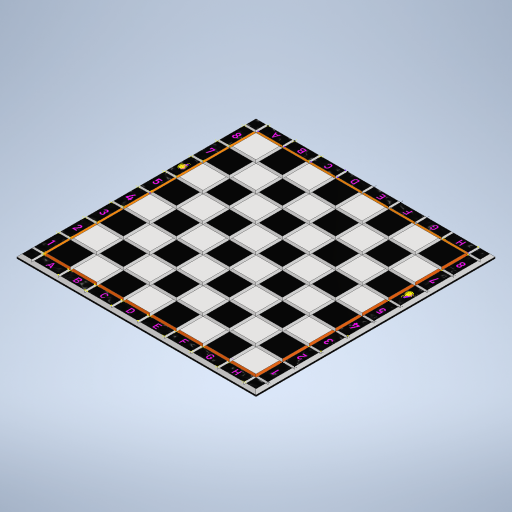
# Autodesk Inventor part: board
Saved by Autodesk Inventor 2024.1 (Build 281209000, 209)
## iProperties
Created: 2025-07-31
Part Number: board
Material: Generic
Document SubType Name: Modeling
Designer: iwheard
Density: 1 g/cm^3
Appearance: Default
Author: iwheard
Autodesk Inventor part; units mm, degrees
(part 1 of 2)
ref_plane "YZ Plane" through (0, 0, 0) normal (1, 0, 0) x (0, 1, 0)
ref_plane "XZ Plane" through (0, 0, 0) normal (0, 1, 0) x (-1, 0, 0)
ref_plane "XY Plane" through (0, 0, 0) normal (0, 0, 1) x (1, 0, 0)
sketch "Sketch1" plane through (0, 0, 0) normal (0, 1, 0) x (-1, 0, 0)
  line L0 (0, 0) -> (-25.5, 0)
  line L1 (-25.5, 0) -> (-25.5, -25.5)
  line L2 (-25.5, -25.5) -> (0, -25.5)
  line L3 (0, -25.5) -> (0, 0)
  dimension "d0" = 25.5
  dimension "d1" = 25.5
  constraints: 8 end point, 2 parallel, 1 horizontal, 1 perpendicular
  measures "d0" distance between parallel lines of L0 L2
  measures "d1" distance between parallel lines of L1 L3
extrude "Extrusion1" add sketch "Sketch1" along normal blind 2.8
chamfer "Chamfer1" distance 1.5 angle 45 4 edges at (12.75, 2.8, 0) (0, 2.8, -12.75) (25.5, 2.8, -12.75) (12.75, 2.8, -25.5)
sketch "Sketch2" plane through (0, 0, 0) normal (0, 1, 0) x (1, 0, 0)
  circle A0 centre (12.75, 12.75) radius 3
  line L0 (0, 0) -> (25.5, 0) projected
  line L1 (25.5, 25.5) -> (0, 25.5) projected
  line L2 (25.5, 0) -> (25.5, 25.5) projected
  line L3 (0, 25.5) -> (0, 0) projected
  dimension "d7" = 6
  dimension "d8" = 25.5
  dimension "d9" = 12.75
  dimension "d10" = 25.5
  dimension "d11" = 12.75
  constraints: 1 centre point
  measures "d7" diameter of A0
  measures "d8" distance between parallel lines of L0 L1
  measures "d9" distance from line of L1 A0.centre
  measures "d10" distance between parallel lines of L2 L3
  measures "d11" distance from line of L2 A0.centre
extrude "Extrusion2" cut sketch "Sketch2" along normal blind 2.5 contours A0
pattern_linear "Rectangular Pattern1" count 8 spacing 25.5 along (1, 0, 0) count 8 spacing 25.5 along (0, 0, -1)
sketch "Sketch5" plane through (0, 0, 0) normal (0, -1, 0) x (1, 0, 0)
  line L0 (0, 0) -> (204, 0) projected
  line L1 (0, -204) -> (0, 0) projected
  line L2 (204, -204) -> (0, -204) projected
  line L3 (204, 0) -> (204, -204) projected
  circle A0 centre (12.75, -38.25) radius 3 projected
  circle A1 centre (38.25, -38.25) radius 3 projected
  circle A2 centre (191.25, -12.75) radius 3 projected
  circle A3 centre (165.75, -12.75) radius 3 projected
  circle A4 centre (140.25, -12.75) radius 3 projected
  circle A5 centre (114.75, -12.75) radius 3 projected
  circle A6 centre (89.25, -12.75) radius 3 projected
  circle A7 centre (63.75, -12.75) radius 3 projected
  circle A8 centre (38.25, -12.75) radius 3 projected
  circle A9 centre (63.75, -38.25) radius 3 projected
  circle A10 centre (89.25, -38.25) radius 3 projected
  circle A11 centre (114.75, -38.25) radius 3 projected
  circle A12 centre (140.25, -38.25) radius 3 projected
  circle A13 centre (165.75, -38.25) radius 3 projected
  circle A14 centre (191.25, -38.25) radius 3 projected
  circle A15 centre (12.75, -63.75) radius 3 projected
  circle A16 centre (38.25, -63.75) radius 3 projected
  circle A17 centre (63.75, -63.75) radius 3 projected
  circle A18 centre (89.25, -63.75) radius 3 projected
  circle A19 centre (114.75, -63.75) radius 3 projected
  circle A20 centre (140.25, -63.75) radius 3 projected
  circle A21 centre (165.75, -63.75) radius 3 projected
  circle A22 centre (191.25, -63.75) radius 3 projected
  circle A23 centre (12.75, -89.25) radius 3 projected
  circle A24 centre (38.25, -89.25) radius 3 projected
  circle A25 centre (63.75, -89.25) radius 3 projected
  circle A26 centre (89.25, -89.25) radius 3 projected
  circle A27 centre (114.75, -89.25) radius 3 projected
  circle A28 centre (140.25, -89.25) radius 3 projected
  circle A29 centre (165.75, -89.25) radius 3 projected
  circle A30 centre (191.25, -89.25) radius 3 projected
  circle A31 centre (12.75, -114.75) radius 3 projected
  circle A32 centre (38.25, -114.75) radius 3 projected
  circle A33 centre (63.75, -114.75) radius 3 projected
  circle A34 centre (89.25, -114.75) radius 3 projected
  circle A35 centre (114.75, -114.75) radius 3 projected
  circle A36 centre (140.25, -114.75) radius 3 projected
  circle A37 centre (165.75, -114.75) radius 3 projected
  circle A38 centre (191.25, -114.75) radius 3 projected
  circle A39 centre (12.75, -140.25) radius 3 projected
  circle A40 centre (38.25, -140.25) radius 3 projected
  circle A41 centre (63.75, -140.25) radius 3 projected
  circle A42 centre (89.25, -140.25) radius 3 projected
  circle A43 centre (114.75, -140.25) radius 3 projected
  circle A44 centre (140.25, -140.25) radius 3 projected
  circle A45 centre (165.75, -140.25) radius 3 projected
  circle A46 centre (191.25, -140.25) radius 3 projected
  circle A47 centre (12.75, -165.75) radius 3 projected
  circle A48 centre (38.25, -165.75) radius 3 projected
  circle A49 centre (63.75, -165.75) radius 3 projected
  circle A50 centre (89.25, -165.75) radius 3 projected
  circle A51 centre (114.75, -165.75) radius 3 projected
  circle A52 centre (140.25, -165.75) radius 3 projected
  circle A53 centre (165.75, -165.75) radius 3 projected
  circle A54 centre (191.25, -165.75) radius 3 projected
  circle A55 centre (12.75, -191.25) radius 3 projected
  circle A56 centre (38.25, -191.25) radius 3 projected
  circle A57 centre (63.75, -191.25) radius 3 projected
  circle A58 centre (89.25, -191.25) radius 3 projected
  circle A59 centre (114.75, -191.25) radius 3 projected
  circle A60 centre (140.25, -191.25) radius 3 projected
  circle A61 centre (165.75, -191.25) radius 3 projected
  circle A62 centre (191.25, -191.25) radius 3 projected
  circle A63 centre (12.75, -12.75) radius 3 projected
  line L4 (0, 0) -> (204, 0) projected
  line L5 (0, -204) -> (0, 0) projected
  line L6 (204, -204) -> (0, -204) projected
  line L7 (204, 0) -> (204, -204) projected
extrude "Extrusion5" add sketch "Sketch5" along normal blind 0.6 separate body
sketch "Sketch6" plane through (0, -0.6, 0) normal (0, -1, 0) x (1, 0, 0)
  line L0 (204, 0) -> (0, 0) projected
  line L1 (0, 0) -> (0, -204) projected
  line L2 (0, -204) -> (204, -204) projected
  line L3 (204, -204) -> (204, 0) projected
  circle A0 centre (191.25, -191.25) radius 3 projected
  circle A1 centre (140.25, -191.25) radius 3 projected
  circle A2 centre (89.25, -191.25) radius 3 projected
  circle A3 centre (38.25, -191.25) radius 3 projected
  circle A4 centre (191.25, -165.75) radius 3 projected
  circle A5 centre (140.25, -165.75) radius 3 projected
  circle A6 centre (89.25, -165.75) radius 3 projected
  circle A7 centre (38.25, -165.75) radius 3 projected
  circle A8 centre (191.25, -140.25) radius 3 projected
  circle A9 centre (140.25, -140.25) radius 3 projected
  circle A10 centre (89.25, -140.25) radius 3 projected
  circle A11 centre (38.25, -140.25) radius 3 projected
  circle A12 centre (191.25, -114.75) radius 3 projected
  circle A13 centre (140.25, -114.75) radius 3 projected
  circle A14 centre (89.25, -114.75) radius 3 projected
  circle A15 centre (38.25, -114.75) radius 3 projected
  circle A16 centre (191.25, -89.25) radius 3 projected
  circle A17 centre (140.25, -89.25) radius 3 projected
  circle A18 centre (89.25, -89.25) radius 3 projected
  circle A19 centre (38.25, -89.25) radius 3 projected
  circle A20 centre (191.25, -63.75) radius 3 projected
  circle A21 centre (140.25, -63.75) radius 3 projected
  circle A22 centre (89.25, -63.75) radius 3 projected
  circle A23 centre (38.25, -63.75) radius 3 projected
  circle A24 centre (191.25, -38.25) radius 3 projected
  circle A25 centre (140.25, -38.25) radius 3 projected
  circle A26 centre (89.25, -38.25) radius 3 projected
  circle A27 centre (38.25, -12.75) radius 3 projected
  circle A28 centre (12.75, -38.25) radius 3 projected
  circle A29 centre (38.25, -38.25) radius 3 projected
  circle A30 centre (191.25, -12.75) radius 3 projected
  circle A31 centre (165.75, -12.75) radius 3 projected
  circle A32 centre (140.25, -12.75) radius 3 projected
  circle A33 centre (114.75, -12.75) radius 3 projected
  circle A34 centre (89.25, -12.75) radius 3 projected
  circle A35 centre (63.75, -12.75) radius 3 projected
  circle A36 centre (63.75, -38.25) radius 3 projected
  circle A37 centre (114.75, -38.25) radius 3 projected
  circle A38 centre (165.75, -38.25) radius 3 projected
  circle A39 centre (12.75, -63.75) radius 3 projected
  circle A40 centre (63.75, -63.75) radius 3 projected
  circle A41 centre (114.75, -63.75) radius 3 projected
  circle A42 centre (165.75, -63.75) radius 3 projected
  circle A43 centre (12.75, -89.25) radius 3 projected
  circle A44 centre (63.75, -89.25) radius 3 projected
  circle A45 centre (114.75, -89.25) radius 3 projected
  circle A46 centre (165.75, -89.25) radius 3 projected
  circle A47 centre (12.75, -114.75) radius 3 projected
  circle A48 centre (63.75, -114.75) radius 3 projected
  circle A49 centre (114.75, -114.75) radius 3 projected
  circle A50 centre (165.75, -114.75) radius 3 projected
  circle A51 centre (12.75, -140.25) radius 3 projected
  circle A52 centre (63.75, -140.25) radius 3 projected
  circle A53 centre (114.75, -140.25) radius 3 projected
  circle A54 centre (165.75, -140.25) radius 3 projected
  circle A55 centre (12.75, -165.75) radius 3 projected
  circle A56 centre (63.75, -165.75) radius 3 projected
  circle A57 centre (114.75, -165.75) radius 3 projected
  circle A58 centre (165.75, -165.75) radius 3 projected
  circle A59 centre (12.75, -191.25) radius 3 projected
  circle A60 centre (63.75, -191.25) radius 3 projected
  circle A61 centre (114.75, -191.25) radius 3 projected
  circle A62 centre (165.75, -191.25) radius 3 projected
  circle A63 centre (12.75, -12.75) radius 3 projected
extrude "Extrusion6" add sketch "Sketch6" along normal blind 1 contours L3 L2 L1 L0 | A0 | A1 | A2 | A3 | A4 | A5 | A6 | A7 | A8 | A9 | A10 | A11 | A12 | A13 | A14 | A15 | A16 | A17 | A18 | A19 | A20 | A21 | A22 | A23 | A24 | A25 | A26 | A27 | A28 | A29 | A30 | A31 | A32 | A33 | A34 | A35 | A36 | A37 | A38 | A39 | A40 | A41 | A42 | A43 | A44 | A45 | A46 | A47 | A48 | A49 | A50 | A51 | A52 | A53 | A54 | A55 | A56 | A57 | A58 | A59 | A60 | A61 | A62 | A63 bodies 2
sketch "Sketch4" plane through (0, -1.6, 0) normal (0, -1, 0) x (1, 0, 0)
  line L0 (0, 0) -> (204, 0) projected
  line L1 (0, -204) -> (0, 0) projected
  line L2 (204, -204) -> (0, -204) projected
  line L3 (204, 0) -> (204, -204) projected
  line L4 (217, 13) -> (-13, 13)
  line L5 (-13, 13) -> (-13, -217)
  line L6 (-13, -217) -> (217, -217)
  line L7 (217, -217) -> (217, 13)
  dimension "d29" = 13
  constraints: 8 end point, 3 other
  measures "d29" distance between parallel lines of L4 L0
extrude "Extrusion4" add sketch "Sketch4" against normal blind 4 bodies 2
chamfer "Chamfer3" distance 1.1 angle 45 4 edges at (0, 2.4, -102) (102, 2.4, -204) (204, 2.4, -102) (102, 2.4, 0)
chamfer "Chamfer4" distance 2.5 angle 45 4 edges at (102, 2.4, 13) (217, 2.4, -102) (102, 2.4, -217) (-13, 2.4, -102)
sketch "Sketch7" plane through (0, 0, 0) normal (0, 1, 0) x (1, 0, 0)
  circle A0 centre (12.75, 12.75) radius 3 projected
  circle A1 centre (12.75, 12.75) radius 3.1
  line L0 (-1.1, -1.1) -> (205.1, -1.1) projected
  line L1 (-1.1, 205.1) -> (-1.1, -1.1) projected
  circle A2 centre (12.75, 38.25) radius 3.1
  circle A3 centre (12.75, 63.75) radius 3.1
  circle A4 centre (12.75, 89.25) radius 3.1
  circle A5 centre (12.75, 114.75) radius 3.1
  circle A6 centre (12.75, 140.25) radius 3.1
  circle A7 centre (12.75, 165.75) radius 3.1
  circle A8 centre (12.75, 191.25) radius 3.1
  circle A9 centre (38.25, 12.75) radius 3.1
  circle A10 centre (38.25, 38.25) radius 3.1
  circle A11 centre (38.25, 63.75) radius 3.1
  circle A12 centre (38.25, 89.25) radius 3.1
  circle A13 centre (38.25, 114.75) radius 3.1
  circle A14 centre (38.25, 140.25) radius 3.1
  circle A15 centre (38.25, 165.75) radius 3.1
  circle A16 centre (38.25, 191.25) radius 3.1
  circle A17 centre (63.75, 12.75) radius 3.1
  circle A18 centre (63.75, 38.25) radius 3.1
  circle A19 centre (63.75, 63.75) radius 3.1
  circle A20 centre (63.75, 89.25) radius 3.1
  circle A21 centre (63.75, 114.75) radius 3.1
  circle A22 centre (63.75, 140.25) radius 3.1
  circle A23 centre (63.75, 165.75) radius 3.1
  circle A24 centre (63.75, 191.25) radius 3.1
  circle A25 centre (89.25, 12.75) radius 3.1
  circle A26 centre (89.25, 38.25) radius 3.1
  circle A27 centre (89.25, 63.75) radius 3.1
  circle A28 centre (89.25, 89.25) radius 3.1
  circle A29 centre (89.25, 114.75) radius 3.1
  circle A30 centre (89.25, 140.25) radius 3.1
  circle A31 centre (89.25, 165.75) radius 3.1
  circle A32 centre (89.25, 191.25) radius 3.1
  circle A33 centre (114.75, 12.75) radius 3.1
  circle A34 centre (114.75, 38.25) radius 3.1
  circle A35 centre (114.75, 63.75) radius 3.1
  circle A36 centre (114.75, 89.25) radius 3.1
  circle A37 centre (114.75, 114.75) radius 3.1
  circle A38 centre (114.75, 140.25) radius 3.1
  circle A39 centre (114.75, 165.75) radius 3.1
  circle A40 centre (114.75, 191.25) radius 3.1
  circle A41 centre (140.25, 12.75) radius 3.1
  circle A42 centre (140.25, 38.25) radius 3.1
  circle A43 centre (140.25, 63.75) radius 3.1
  circle A44 centre (140.25, 89.25) radius 3.1
  circle A45 centre (140.25, 114.75) radius 3.1
  circle A46 centre (140.25, 140.25) radius 3.1
  circle A47 centre (140.25, 165.75) radius 3.1
  circle A48 centre (140.25, 191.25) radius 3.1
  circle A49 centre (165.75, 12.75) radius 3.1
  circle A50 centre (165.75, 38.25) radius 3.1
  circle A51 centre (165.75, 63.75) radius 3.1
  circle A52 centre (165.75, 89.25) radius 3.1
  circle A53 centre (165.75, 114.75) radius 3.1
  circle A54 centre (165.75, 140.25) radius 3.1
  circle A55 centre (165.75, 165.75) radius 3.1
  circle A56 centre (165.75, 191.25) radius 3.1
  circle A57 centre (191.25, 12.75) radius 3.1
  circle A58 centre (191.25, 38.25) radius 3.1
  circle A59 centre (191.25, 63.75) radius 3.1
  circle A60 centre (191.25, 89.25) radius 3.1
  circle A61 centre (191.25, 114.75) radius 3.1
  circle A62 centre (191.25, 140.25) radius 3.1
  circle A63 centre (191.25, 165.75) radius 3.1
  circle A64 centre (191.25, 191.25) radius 3.1
  point P0 (0, 0)
  dimension "d42" = 0.1
  dimension "d45" = 25.5
  dimension "d48" = 25.5
  constraints: 64 centre point, 1 horizontal, 1 vertical, 126 other
  measures "d42" radial gap between concentric circles of A1 A0
  measures "d45" distance of A0.centre A2.centre
  measures "d48" distance of A0.centre A9.centre
extrude "Extrusion7" cut sketch "Sketch7" against normal blind 0.6 bodies 2
sketch "Sketch8" plane through (-13, -1.6, 13) normal (0, 0, 1) x (1, 0, 0)
  line L0 (37, 4.4) -> (38.5, 2.9) projected
  line L1 (40, 4.4) -> (38.5, 2.9) projected
  line L2 (37, 4.4) -> (14.5, 4.4) projected
  line L3 (14.5, 4.4) -> (13, 2.9) projected
  line L4 (13, 2.9) -> (38.5, 2.9) projected
  line L5 (38.5, 2.9) -> (64, 2.9) projected
  line L6 (62.5, 4.4) -> (64, 2.9) projected
  line L7 (65.5, 4.4) -> (64, 2.9) projected
  line L8 (88, 4.4) -> (65.5, 4.4) projected
  line L9 (64, 2.9) -> (89.5, 2.9) projected
  line L10 (88, 4.4) -> (89.5, 2.9) projected
  line L11 (91, 4.4) -> (89.5, 2.9) projected
  line L12 (89.5, 2.9) -> (115, 2.9) projected
  line L13 (113.5, 4.4) -> (91, 4.4) projected
  line L14 (113.5, 4.4) -> (115, 2.9) projected
  line L15 (116.5, 4.4) -> (115, 2.9) projected
  line L16 (139, 4.4) -> (116.5, 4.4) projected
  line L17 (115, 2.9) -> (140.5, 2.9) projected
  line L18 (139, 4.4) -> (140.5, 2.9) projected
  line L19 (142, 4.4) -> (140.5, 2.9) projected
  line L20 (164.5, 4.4) -> (142, 4.4) projected
  line L21 (140.5, 2.9) -> (166, 2.9) projected
  line L22 (164.5, 4.4) -> (166, 2.9) projected
  line L23 (167.5, 4.4) -> (166, 2.9) projected
  line L24 (190, 4.4) -> (167.5, 4.4) projected
  line L25 (166, 2.9) -> (191.5, 2.9) projected
  line L26 (190, 4.4) -> (191.5, 2.9) projected
  line L27 (193, 4.4) -> (191.5, 2.9) projected
  line L28 (191.5, 2.9) -> (217, 2.9) projected
  line L29 (215.5, 4.4) -> (193, 4.4) projected
  line L30 (215.5, 4.4) -> (217, 2.9) projected
  line L31 (62.5, 4.4) -> (40, 4.4) projected
  line L32 (37, 4.4) -> (193, 4.4)
  line L33 (2.5, 4) -> (227.5, 4) projected
  line L34 (11.9, 4) -> (13, 2.9) projected
  line L35 (218.1, 4) -> (217, 2.9) projected
  point P0 (13, 1.6)
  point P1 (13, 2.9)
  point P2 (14.1, 4)
  point P3 (39.6, 4)
  point P4 (37.4, 4)
  point P5 (65.1, 4)
  point P6 (62.9, 4)
  point P7 (90.6, 4)
  point P8 (88.4, 4)
  point P9 (116.1, 4)
  point P10 (113.9, 4)
  point P11 (141.6, 4)
  point P12 (139.4, 4)
  point P13 (167.1, 4)
  point P14 (164.9, 4)
  point P15 (190, 4.4)
  point P16 (215.9, 4)
  constraints: 2 end point, 1 parallel
extrude "Extrusion8" cut sketch "Sketch8" along normal through all both and the other way through all contours L33 L1 L0 | L3 L34 L33 | L6 L33 L7 | L10 L33 L11 | L14 L33 L15 | L18 L33 L19 | L22 L33 L23 | L26 L33 L27 | L26 L32 L27 L33 | L30 L33 L35 bodies 2
sketch "Sketch9" plane through (-13, -1.6, -217) normal (-1, 0, 0) x (0, 0, 1)
  line L0 (13, 2.9) -> (38.5, 2.9) projected
  line L1 (37, 4.4) -> (38.5, 2.9) projected
  line L2 (37, 4.4) -> (14.5, 4.4) projected
  line L3 (14.5, 4.4) -> (13, 2.9) projected
  line L4 (38.5, 2.9) -> (64, 2.9) projected
  line L5 (62.5, 4.4) -> (64, 2.9) projected
  line L6 (62.5, 4.4) -> (40, 4.4) projected
  line L7 (40, 4.4) -> (38.5, 2.9) projected
  line L8 (64, 2.9) -> (89.5, 2.9) projected
  line L9 (88, 4.4) -> (89.5, 2.9) projected
  line L10 (88, 4.4) -> (65.5, 4.4) projected
  line L11 (65.5, 4.4) -> (64, 2.9) projected
  line L12 (89.5, 2.9) -> (115, 2.9) projected
  line L13 (113.5, 4.4) -> (115, 2.9) projected
  line L14 (113.5, 4.4) -> (91, 4.4) projected
  line L15 (91, 4.4) -> (89.5, 2.9) projected
  line L16 (139, 4.4) -> (116.5, 4.4) projected
  line L17 (115, 2.9) -> (140.5, 2.9) projected
  line L18 (139, 4.4) -> (140.5, 2.9) projected
  line L19 (139, 4.4) -> (116.5, 4.4) projected
  line L20 (116.5, 4.4) -> (115, 2.9) projected
  line L21 (227.5, 4) -> (2.5, 4) projected
  line L22 (140.5, 2.9) -> (166, 2.9) projected
  line L23 (164.5, 4.4) -> (166, 2.9) projected
  line L24 (164.5, 4.4) -> (142, 4.4) projected
  line L25 (142, 4.4) -> (140.5, 2.9) projected
  line L26 (166, 2.9) -> (191.5, 2.9) projected
  line L27 (190, 4.4) -> (191.5, 2.9) projected
  line L28 (190, 4.4) -> (167.5, 4.4) projected
  line L29 (167.5, 4.4) -> (166, 2.9) projected
  line L30 (191.5, 2.9) -> (217, 2.9) projected
  line L31 (215.5, 4.4) -> (217, 2.9) projected
  line L32 (215.5, 4.4) -> (193, 4.4) projected
  line L33 (193, 4.4) -> (191.5, 2.9) projected
  line L34 (217, 2.9) -> (217, 2.9) projected
  line L35 (0, 1.5) -> (230, 1.5) projected
  line L36 (227.5, 4) -> (230, 1.5) projected
  line L37 (227.5, 4) -> (2.5, 4) projected
  line L38 (2.5, 4) -> (0, 1.5) projected
  line L39 (11.9, 4) -> (13, 2.9) projected
  line L40 (217, 2.9) -> (218.1, 4) projected
  point P0 (217, 1.6)
  point P1 (215.9, 4)
  point P2 (192.6, 4)
  point P3 (190.4, 4)
  point P4 (167.1, 4)
  point P5 (164.9, 4)
  point P6 (141.6, 4)
  point P7 (139.4, 4)
  point P8 (116.1, 4)
  point P9 (113.9, 4)
  point P10 (90.6, 4)
  point P11 (88.4, 4)
  point P12 (65.1, 4)
  point P13 (62.9, 4)
  point P14 (39.6, 4)
  point P15 (37.4, 4)
  point P16 (14.1, 4)
  constraints: 2 other
extrude "Extrusion9" cut sketch "Sketch9" along normal through all both and the other way through all contours L39 L21 L3 | L1 L21 L7 | L5 L21 L11 | L9 L21 L15 | L13 L21 L20 | L18 L21 L25 | L23 L21 L29 | L40 L31 L21 | L27 L21 L33 | L21 L33 L32 L31 bodies 2
sketch "Sketch10" plane through (0, 2.4, 0) normal (0, 1, 0) x (1, 0, 0)
  line L0 (-10.5, 24.4) -> (-1.1, 24.4) construction
  line L1 (-1.1, 24.4) -> (-1.1, 1.1) construction
  line L2 (-1.1, 1.1) -> (-10.5, 1.1) construction
  line L3 (-10.5, 1.1) -> (-10.5, 24.4) construction
  line L4 (1.1, -1.1) -> (24.4, -1.1) construction
  line L5 (24.4, -1.1) -> (24.4, -10.5) construction
  line L6 (24.4, -10.5) -> (1.1, -10.5) construction
  line L7 (1.1, -10.5) -> (1.1, -1.1) construction
  line L8 (26.6, -10.5) -> (26.6, -1.1) construction
  line L9 (26.6, -1.1) -> (49.9, -1.1) construction
  line L10 (49.9, -1.1) -> (49.9, -10.5) construction
  line L11 (49.9, -10.5) -> (26.6, -10.5) construction
  line L12 (52.1, -10.5) -> (52.1, -1.1) construction
  line L13 (52.1, -1.1) -> (75.4, -1.1) construction
  line L14 (75.4, -1.1) -> (75.4, -10.5) construction
  line L15 (75.4, -10.5) -> (52.1, -10.5) construction
  line L16 (77.6, -10.5) -> (77.6, -1.1) construction
  line L17 (77.6, -1.1) -> (100.9, -1.1) construction
  line L18 (100.9, -1.1) -> (100.9, -10.5) construction
  line L19 (100.9, -10.5) -> (77.6, -10.5) construction
  line L20 (103.1, -10.5) -> (103.1, -1.1) construction
  line L21 (103.1, -1.1) -> (126.4, -1.1) construction
  line L22 (126.4, -1.1) -> (126.4, -10.5) construction
  line L23 (126.4, -10.5) -> (103.1, -10.5) construction
  line L24 (128.6, -10.5) -> (128.6, -1.1) construction
  line L25 (128.6, -1.1) -> (151.9, -1.1) construction
  line L26 (151.9, -1.1) -> (151.9, -10.5) construction
  line L27 (151.9, -10.5) -> (128.6, -10.5) construction
  line L28 (154.1, -10.5) -> (154.1, -1.1) construction
  line L29 (154.1, -1.1) -> (177.4, -1.1) construction
  line L30 (177.4, -1.1) -> (177.4, -10.5) construction
  line L31 (177.4, -10.5) -> (154.1, -10.5) construction
  line L32 (179.6, -10.5124) -> (179.6, -1.1) construction
  line L33 (179.6, -1.1) -> (202.9, -1.1) construction
  line L34 (202.9, -1.1) -> (202.9, -10.5124) construction
  line L35 (202.9, -10.5124) -> (179.6, -10.5124) construction
  line L36 (-10.5, 49.9) -> (-1.1, 49.9) construction
  line L37 (-1.1, 49.9) -> (-1.1, 26.6) construction
  line L38 (-1.1, 26.6) -> (-10.5, 26.6) construction
  line L39 (-10.5, 26.6) -> (-10.5, 49.9) construction
  line L40 (-10.5, 75.4) -> (-1.1, 75.4) construction
  line L41 (-1.1, 75.4) -> (-1.1, 52.1) construction
  line L42 (-1.1, 52.1) -> (-10.5, 52.1) construction
  line L43 (-10.5, 52.1) -> (-10.5, 75.4) construction
  line L44 (-10.5, 77.6) -> (-10.5, 100.9) construction
  line L45 (-10.5, 100.9) -> (-1.1, 100.9) construction
  line L46 (-1.1, 100.9) -> (-1.1, 77.6) construction
  line L47 (-1.1, 77.6) -> (-10.5, 77.6) construction
  line L48 (-10.5, 126.4) -> (-1.1, 126.4) construction
  line L49 (-1.1, 126.4) -> (-1.1, 103.1) construction
  line L50 (-1.1, 103.1) -> (-10.5, 103.1) construction
  line L51 (-10.5, 103.1) -> (-10.5, 126.4) construction
  line L52 (-10.5, 128.6) -> (-10.5, 151.9) construction
  line L53 (-10.5, 151.9) -> (-1.1, 151.9) construction
  line L54 (-1.1, 151.9) -> (-1.1, 128.6) construction
  line L55 (-1.1, 128.6) -> (-10.5, 128.6) construction
  line L56 (-10.5, 179.6) -> (-10.5, 202.9) construction
  line L57 (-10.5, 202.9) -> (-1.1, 202.9) construction
  line L58 (-1.1, 202.9) -> (-1.1, 179.6) construction
  line L59 (-1.1, 179.6) -> (-10.5, 179.6) construction
  line L60 (-10.5, 154.1) -> (-10.5, 177.4) construction
  line L61 (-10.5, 177.4) -> (-1.1, 177.4) construction
  line L62 (-1.1, 177.4) -> (-1.1, 154.1) construction
  line L63 (-1.1, 154.1) -> (-10.5, 154.1) construction
  line L64 (214.5, 1.1) -> (205.1, 1.1) construction
  line L65 (205.1, 1.1) -> (205.1, 24.4) construction
  line L66 (205.1, 24.4) -> (214.5, 24.4) construction
  line L67 (214.5, 24.4) -> (214.5, 1.1) construction
  line L68 (24.4, 214.5) -> (24.4, 205.1) construction
  line L69 (24.4, 205.1) -> (1.1, 205.1) construction
  line L70 (1.1, 205.1) -> (1.1, 214.5) construction
  line L71 (1.1, 214.5) -> (24.4, 214.5) construction
  line L72 (49.9, 214.5) -> (49.9, 205.1) construction
  line L73 (49.9, 205.1) -> (26.6, 205.1) construction
  line L74 (26.6, 205.1) -> (26.6, 214.5) construction
  line L75 (26.6, 214.5) -> (49.9, 214.5) construction
  line L76 (75.4, 214.5) -> (75.4, 205.1) construction
  line L77 (75.4, 205.1) -> (52.1, 205.1) construction
  line L78 (52.1, 205.1) -> (52.1, 214.5) construction
  line L79 (52.1, 214.5) -> (75.4, 214.5) construction
  line L80 (100.9, 214.5) -> (100.9, 205.1) construction
  line L81 (100.9, 205.1) -> (77.6, 205.1) construction
  line L82 (77.6, 205.1) -> (77.6, 214.5) construction
  line L83 (77.6, 214.5) -> (100.9, 214.5) construction
  line L84 (151.9, 214.5) -> (151.9, 205.1) construction
  line L85 (151.9, 205.1) -> (128.6, 205.1) construction
  line L86 (128.6, 205.1) -> (128.6, 214.5) construction
  line L87 (128.6, 214.5) -> (151.9, 214.5) construction
  line L88 (126.4, 214.5) -> (126.4, 205.1) construction
  line L89 (126.4, 205.1) -> (103.1, 205.1) construction
  line L90 (103.1, 205.1) -> (103.1, 214.5) construction
  line L91 (103.1, 214.5) -> (126.4, 214.5) construction
  line L92 (202.9, 214.5) -> (202.9, 205.1) construction
  line L93 (202.9, 205.1) -> (179.6, 205.1) construction
  line L94 (179.6, 205.1) -> (179.6, 214.5) construction
  line L95 (179.6, 214.5) -> (202.9, 214.5) construction
  line L96 (177.4, 214.5) -> (177.4, 205.1) construction
  line L97 (177.4, 205.1) -> (154.1, 205.1) construction
  line L98 (154.1, 205.1) -> (154.1, 214.5) construction
  line L99 (154.1, 214.5) -> (177.4, 214.5) construction
  line L100 (214.5, 49.9) -> (214.5, 26.6) construction
  line L101 (214.5, 26.6) -> (205.1, 26.6) construction
  line L102 (205.1, 26.6) -> (205.1, 49.9) construction
  line L103 (205.1, 49.9) -> (214.5, 49.9) construction
  line L104 (214.5, 100.9) -> (214.5, 77.6) construction
  line L105 (214.5, 77.6) -> (205.1, 77.6) construction
  line L106 (205.1, 77.6) -> (205.1, 100.9) construction
  line L107 (205.1, 100.9) -> (214.5, 100.9) construction
  line L108 (214.5, 75.4) -> (214.5, 52.1) construction
  line L109 (214.5, 52.1) -> (205.1, 52.1) construction
  line L110 (205.1, 52.1) -> (205.1, 75.4) construction
  line L111 (205.1, 75.4) -> (214.5, 75.4) construction
  line L112 (214.5, 177.4) -> (214.5, 154.1) construction
  line L113 (214.5, 154.1) -> (205.1, 154.1) construction
  line L114 (205.1, 154.1) -> (205.1, 177.4) construction
  line L115 (205.1, 177.4) -> (214.5, 177.4) construction
  line L116 (214.5, 202.9) -> (214.5, 179.6) construction
  line L117 (214.5, 179.6) -> (205.1, 179.6) construction
  line L118 (205.1, 179.6) -> (205.1, 202.9) construction
  line L119 (205.1, 202.9) -> (214.5, 202.9) construction
  line L120 (214.5, 151.9) -> (214.5, 128.6) construction
  line L121 (214.5, 128.6) -> (205.1, 128.6) construction
  line L122 (205.1, 128.6) -> (205.1, 151.9) construction
  line L123 (205.1, 151.9) -> (214.5, 151.9) construction
  line L124 (214.5, 126.4) -> (214.5, 103.1) construction
  line L125 (214.5, 103.1) -> (205.1, 103.1) construction
  line L126 (205.1, 103.1) -> (205.1, 126.4) construction
  line L127 (205.1, 126.4) -> (214.5, 126.4) construction
  line L128 (-5.8517, 143.7982) -> (-4.5401, 143.7982) construction
  line L129 (-4.5401, 143.7982) -> (-4.5134, 143.8343) construction
  line L130 (-4.5134, 143.8343) -> (-4.5585, 143.7444) construction
  line L131 (-4.5585, 143.7444) -> (-5.9824, 140.9055) construction
  line L132 (-5.9824, 140.9055) -> (-5.9824, 140.8854) construction
  line L133 (-5.9824, 140.8854) -> (-5.9205, 140.9095) construction
  line L134 (-5.9205, 140.9095) -> (-5.7874, 140.9496) construction
  line L135 (-5.7874, 140.9496) -> (-5.2793, 140.9365) construction
  line L136 (-5.2793, 140.9365) -> (-5.183, 140.919) construction
  line L137 (-5.183, 140.919) -> (-4.3467, 140.7069) construction
  line L138 (-5.872, 136.6416) -> (-6.371, 136.7634) construction
  line L139 (-7.5664, 140.3415) -> (-5.8517, 143.7982) construction
  spline S0 degree 4 poles (-5.8517, 143.7982) (-4.5401, 143.7982) (-4.5134, 143.8343) (-4.5585, 143.7444) (-5.9824, 140.9055) (-5.9824, 140.8854) (-5.9205, 140.9095) (-5.7874, 140.9496) (-5.2793, 140.9365) (-5.183, 140.919) (-4.3467, 140.7069) (-3.7965, 139.7773) (-3.7431, 138.3045) (-4.0298, 137.6549) (-4.2865, 137.2661) (-4.7485, 136.8027) (-5.872, 136.6416) (-6.371, 136.7634) (-6.95, 136.8756) (-7.681, 137.6176) (-7.8548, 138.6944) (-7.7494, 139.6846) (-7.5664, 140.3415) (-5.8517, 143.7982) knots 0 0 0 0 0 1 2 3 4 5 6 7 8 9 10 11 12 13 14 15 16 17 18 19 20 20 20 20 20
  line L140 (-5.9044, 139.8261) -> (-5.5333, 139.8261) construction
  line L141 (-5.5333, 139.8261) -> (-5.3147, 139.705) construction
  line L142 (-5.3147, 139.705) -> (-4.9281, 139.3692) construction
  line L143 (-4.9281, 139.3692) -> (-4.9552, 138.4359) construction
  line L144 (-4.9552, 138.4359) -> (-5.1249, 138.0303) construction
  line L145 (-5.1249, 138.0303) -> (-5.5713, 137.7938) construction
  line L146 (-5.5713, 137.7938) -> (-6.105, 137.831) construction
  line L147 (-6.105, 137.831) -> (-6.6109, 138.1387) construction
  line L148 (-6.6109, 138.1387) -> (-6.6605, 138.8752) construction
  line L149 (-6.6605, 138.8752) -> (-6.5478, 139.4625) construction
  line L150 (-6.5478, 139.4625) -> (-6.2798, 139.7445) construction
  line L151 (-6.2798, 139.7445) -> (-5.9044, 139.8261) construction
  spline S1 degree 4 poles (-5.9044, 139.8261) (-5.5333, 139.8261) (-5.3147, 139.705) (-4.9281, 139.3692) (-4.9552, 138.4359) (-5.1249, 138.0303) (-5.5713, 137.7938) (-6.105, 137.831) (-6.6109, 138.1387) (-6.6605, 138.8752) (-6.5478, 139.4625) (-6.2798, 139.7445) (-5.9044, 139.8261) knots 1 1 1 1 1 2 3 4 5 6 7 8 9 10 10 10 10 10
  line L152 (-7.8548, 138.6944) -> (-7.7494, 139.6846) construction
  line L153 (-7.7494, 139.6846) -> (-7.5664, 140.3415) construction
  line L154 (-6.371, 136.7634) -> (-6.95, 136.8756) construction
  line L155 (-6.95, 136.8756) -> (-7.681, 137.6176) construction
  line L156 (-7.681, 137.6176) -> (-7.8548, 138.6944) construction
  line L157 (-4.2865, 137.2661) -> (-4.7485, 136.8027) construction
  line L158 (-4.7485, 136.8027) -> (-5.872, 136.6416) construction
  line L159 (-4.3467, 140.7069) -> (-3.7965, 139.7773) construction
  line L160 (-3.7965, 139.7773) -> (-3.7431, 138.3045) construction
  line L161 (-3.7431, 138.3045) -> (-4.0298, 137.6549) construction
  line L162 (-4.0298, 137.6549) -> (-4.2865, 137.2661) construction
  line L163 (209.8269, 136.6677) -> (208.5153, 136.6677) construction
  line L164 (208.5153, 136.6677) -> (208.4886, 136.6317) construction
  line L165 (208.4886, 136.6317) -> (208.5337, 136.7215) construction
  line L166 (208.5337, 136.7215) -> (209.9576, 139.5604) construction
  line L167 (209.9576, 139.5604) -> (209.9576, 139.5806) construction
  line L168 (209.9576, 139.5806) -> (209.8957, 139.5564) construction
  line L169 (209.8957, 139.5564) -> (209.7626, 139.5163) construction
  line L170 (209.7626, 139.5163) -> (209.2545, 139.5294) construction
  line L171 (209.2545, 139.5294) -> (209.1582, 139.5469) construction
  line L172 (209.1582, 139.5469) -> (208.3219, 139.7591) construction
  line L173 (209.8472, 143.8243) -> (210.3462, 143.7026) construction
  line L174 (211.5416, 140.1244) -> (209.8269, 136.6677) construction
  spline S2 degree 4 poles (209.8269, 136.6677) (208.5153, 136.6677) (208.4886, 136.6317) (208.5337, 136.7215) (209.9576, 139.5604) (209.9576, 139.5806) (209.8957, 139.5564) (209.7626, 139.5163) (209.2545, 139.5294) (209.1582, 139.5469) (208.3219, 139.7591) (207.7717, 140.6886) (207.7183, 142.1614) (208.005, 142.8111) (208.2617, 143.1999) (208.7237, 143.6632) (209.8472, 143.8243) (210.3462, 143.7026) (210.9252, 143.5904) (211.6562, 142.8483) (211.83, 141.7715) (211.7246, 140.7813) (211.5416, 140.1244) (209.8269, 136.6677) knots 0 0 0 0 0 1 2 3 4 5 6 7 8 9 10 11 12 13 14 15 16 17 18 19 20 20 20 20 20
  line L175 (209.8796, 140.6399) -> (209.5085, 140.6399) construction
  line L176 (209.5085, 140.6399) -> (209.2899, 140.7609) construction
  line L177 (209.2899, 140.7609) -> (208.9033, 141.0967) construction
  line L178 (208.9033, 141.0967) -> (208.9304, 142.03) construction
  line L179 (208.9304, 142.03) -> (209.1001, 142.4356) construction
  line L180 (209.1001, 142.4356) -> (209.5465, 142.6722) construction
  line L181 (209.5465, 142.6722) -> (210.0802, 142.6349) construction
  line L182 (210.0802, 142.6349) -> (210.5861, 142.3272) construction
  line L183 (210.5861, 142.3272) -> (210.6357, 141.5908) construction
  line L184 (210.6357, 141.5908) -> (210.523, 141.0035) construction
  line L185 (210.523, 141.0035) -> (210.255, 140.7215) construction
  line L186 (210.255, 140.7215) -> (209.8796, 140.6399) construction
  spline S3 degree 4 poles (209.8796, 140.6399) (209.5085, 140.6399) (209.2899, 140.7609) (208.9033, 141.0967) (208.9304, 142.03) (209.1001, 142.4356) (209.5465, 142.6722) (210.0802, 142.6349) (210.5861, 142.3272) (210.6357, 141.5908) (210.523, 141.0035) (210.255, 140.7215) (209.8796, 140.6399) knots 1 1 1 1 1 2 3 4 5 6 7 8 9 10 10 10 10 10
  line L187 (211.83, 141.7715) -> (211.7246, 140.7813) construction
  line L188 (211.7246, 140.7813) -> (211.5416, 140.1244) construction
  line L189 (210.3462, 143.7026) -> (210.9252, 143.5904) construction
  line L190 (210.9252, 143.5904) -> (211.6562, 142.8483) construction
  line L191 (211.6562, 142.8483) -> (211.83, 141.7715) construction
  line L192 (208.2617, 143.1999) -> (208.7237, 143.6632) construction
  line L193 (208.7237, 143.6632) -> (209.8472, 143.8243) construction
  line L194 (208.3219, 139.7591) -> (207.7717, 140.6886) construction
  line L195 (207.7717, 140.6886) -> (207.7183, 142.1614) construction
  line L196 (207.7183, 142.1614) -> (208.005, 142.8111) construction
  line L197 (208.005, 142.8111) -> (208.2617, 143.1999) construction
  line L198 (15.4071, 212.85) -> (13.1152, 206.75)
  line L199 (13.1152, 206.75) -> (12.3848, 206.75)
  line L200 (12.3848, 206.75) -> (10.0929, 212.85)
  line L201 (10.0929, 212.85) -> (11.1709, 212.85)
  line L202 (11.1709, 212.85) -> (12.7525, 208.3065)
  line L203 (12.7525, 208.3065) -> (14.3241, 212.85)
  line L204 (14.3241, 212.85) -> (15.4071, 212.85)
  line L205 (14.3291, 211.6915) -> (14.3291, 210.7294)
  line L206 (14.3291, 210.7294) -> (11.1205, 210.7294)
  line L207 (11.1205, 210.7294) -> (11.1205, 211.6915)
  line L208 (11.1205, 211.6915) -> (14.3291, 211.6915)
  line L209 (39.804, 212.85) -> (39.804, 211.898)
  line L210 (39.804, 211.898) -> (38.0057, 211.898)
  spline S4 degree 2 poles (38.0057, 211.898) (37.4667, 211.898) (36.968, 211.4497) (36.968, 211.0618) knots 0 0 0 1 2 2 2
  line L211 (36.968, 211.0618) -> (36.968, 211.0517)
  spline S5 degree 2 poles (36.968, 211.0517) (36.968, 210.6488) (37.4264, 210.1904) (37.8999, 210.1904) knots 0 0 0 1 2 2 2
  line L212 (37.8999, 210.1904) -> (39.804, 210.1904)
  line L213 (39.804, 210.1904) -> (39.804, 209.2484)
  line L214 (39.804, 209.2484) -> (37.8999, 209.2484)
  spline S6 degree 2 poles (37.8999, 209.2484) (37.4869, 209.2484) (37.0486, 208.8404) (37.0486, 208.4626) knots 0 0 0 1 2 2 2
  spline S7 degree 2 poles (37.0486, 208.4626) (37.0486, 208.0899) (37.5121, 207.697) (37.9604, 207.697) knots 0 0 0 1 2 2 2
  line L215 (37.9604, 207.697) -> (39.804, 207.697)
  line L216 (39.804, 207.697) -> (39.804, 206.75)
  line L217 (39.804, 206.75) -> (37.8647, 206.75)
  spline S8 degree 2 poles (37.8647, 206.75) (36.963, 206.75) (36.0362, 207.6315) (36.0362, 208.4022) knots 0 0 0 1 2 2 2
  spline S9 degree 2 poles (36.0362, 208.4022) (36.0362, 208.8958) (36.6154, 209.6212) (37.1897, 209.7219) knots 0 0 0 1 2 2 2
  spline S10 degree 2 poles (37.1897, 209.7219) (36.6054, 209.8076) (35.9606, 210.5984) (35.9606, 211.1777) knots 0 0 0 1 2 2 2
  line L218 (35.9606, 211.1777) -> (35.9606, 211.1877)
  spline S11 degree 2 poles (35.9606, 211.1877) (35.9606, 211.9584) (36.9328, 212.85) (37.7941, 212.85) knots 0 0 0 1 2 2 2
  line L219 (37.7941, 212.85) -> (39.804, 212.85)
  line L220 (40.3077, 212.85) -> (40.3077, 206.75)
  line L221 (40.3077, 206.75) -> (39.3053, 206.75)
  line L222 (39.3053, 206.75) -> (39.3053, 212.85)
  line L223 (39.3053, 212.85) -> (40.3077, 212.85)
  spline S12 degree 2 poles (-5.8, 187.6806) (-6.4532, 187.6806) (-7.4301, 188.1604) (-7.9734, 189.0332) (-7.9734, 189.6228) knots 0 0 0 1 2 3 3 3
  line L224 (-7.9734, 189.6228) -> (-7.9734, 189.7384)
  spline S13 degree 2 poles (-7.9734, 189.7384) (-7.9734, 190.2645) (-7.4185, 191.1893) (-6.9618, 191.4263) knots 0 0 0 1 2 2 2
  spline S14 degree 2 poles (-6.9618, 191.4263) (-7.3491, 191.6286) (-7.8289, 192.3858) (-7.8289, 192.8078) knots 0 0 0 1 2 2 2
  line L225 (-7.8289, 192.8078) -> (-7.8289, 192.9812)
  spline S15 degree 2 poles (-7.8289, 192.9812) (-7.8289, 193.8194) (-6.7133, 194.8251) (-5.8, 194.8251) knots 0 0 0 1 2 2 2
  spline S16 degree 2 poles (-5.8, 194.8251) (-4.8867, 194.8251) (-3.7711, 193.8194) (-3.7711, 192.9812) knots 0 0 0 1 2 2 2
  line L226 (-3.7711, 192.9812) -> (-3.7711, 192.8078)
  spline S17 degree 2 poles (-3.7711, 192.8078) (-3.7711, 192.3801) (-4.2566, 191.6228) (-4.6555, 191.4263) knots 0 0 0 1 2 2 2
  spline S18 degree 2 poles (-4.6555, 191.4263) (-4.1931, 191.1893) (-3.6266, 190.2645) (-3.6266, 189.7384) knots 0 0 0 1 2 2 2
  line L227 (-3.6266, 189.7384) -> (-3.6266, 189.6228)
  spline S19 degree 2 poles (-3.6266, 189.6228) (-3.6266, 189.0332) (-4.1757, 188.1604) (-5.1468, 187.6806) (-5.8, 187.6806) knots 0 0 0 1 2 3 3 3
  spline S20 degree 2 poles (-5.8, 188.7847) (-5.3376, 188.7847) (-4.7769, 189.3223) (-4.7769, 189.7558) knots 0 0 0 1 2 2 2
  line L228 (-4.7769, 189.7558) -> (-4.7769, 189.8251)
  spline S21 degree 2 poles (-4.7769, 189.8251) (-4.7769, 190.2471) (-5.3376, 190.7616) (-5.8, 190.7616) knots 0 0 0 1 2 2 2
  spline S22 degree 2 poles (-5.8, 190.7616) (-6.2566, 190.7616) (-6.8289, 190.2471) (-6.8231, 189.8194) knots 0 0 0 1 2 2 2
  line L229 (-6.8231, 189.8194) -> (-6.8231, 189.75)
  spline S23 degree 2 poles (-6.8231, 189.75) (-6.8231, 189.3165) (-6.2624, 188.7847) (-5.8, 188.7847) knots 0 0 0 1 2 2 2
  spline S24 degree 2 poles (-5.8, 191.8656) (-5.4069, 191.8714) (-4.9272, 192.3743) (-4.9272, 192.7847) knots 0 0 0 1 2 2 2
  line L230 (-4.9272, 192.7847) -> (-4.9272, 192.854)
  spline S25 degree 2 poles (-4.9272, 192.854) (-4.9272, 193.2413) (-5.4069, 193.7153) (-5.8, 193.7153) knots 0 0 0 1 2 2 2
  spline S26 degree 2 poles (-5.8, 193.7153) (-6.1931, 193.7153) (-6.6786, 193.2413) (-6.6786, 192.8483) knots 0 0 0 1 2 2 2
  line L231 (-6.6786, 192.8483) -> (-6.6786, 192.7789)
  spline S27 degree 2 poles (-6.6786, 192.7789) (-6.6786, 192.3627) (-6.1931, 191.8656) (-5.8, 191.8656) knots 0 0 0 1 2 2 2
  line L232 (-3.8954, 169.25) -> (-3.8954, 168.3772)
  line L233 (-3.8954, 168.3772) -> (-5.589, 162.25)
  line L234 (-5.589, 162.25) -> (-6.826, 162.25)
  line L235 (-6.826, 162.25) -> (-5.1555, 168.146)
  line L236 (-5.1555, 168.146) -> (-6.6526, 168.146)
  line L237 (-6.6526, 168.146) -> (-6.6526, 167.1171)
  line L238 (-6.6526, 167.1171) -> (-7.8029, 167.1171)
  line L239 (-7.8029, 167.1171) -> (-7.8029, 169.25)
  line L240 (-7.8029, 169.25) -> (-3.8954, 169.25)
  spline S28 degree 2 poles (-5.8087, 111.2182) (-6.6237, 111.2182) (-7.7104, 112.224) (-7.8087, 113.1373) knots 0 0 0 1 2 2 2
  line L241 (-7.8087, 113.1373) -> (-7.8087, 113.1488)
  line L242 (-7.8087, 113.1488) -> (-6.6584, 113.1488)
  line L243 (-6.6584, 113.1488) -> (-6.6584, 113.1431)
  spline S29 degree 2 poles (-6.6584, 113.1431) (-6.6179, 112.7558) (-6.1613, 112.328) (-5.7971, 112.328) knots 0 0 0 1 2 2 2
  spline S30 degree 2 poles (-5.7971, 112.328) (-5.3867, 112.328) (-4.9416, 112.8714) (-4.9416, 113.3627) knots 0 0 0 1 2 2 2
  line L244 (-4.9416, 113.3627) -> (-4.9416, 113.9523)
  spline S31 degree 2 poles (-4.9416, 113.9523) (-4.9416, 114.4436) (-5.3636, 114.9812) (-5.7624, 114.9812) knots 0 0 0 1 2 2 2
  spline S32 degree 2 poles (-5.7624, 114.9812) (-6.0283, 114.9812) (-6.4618, 114.6922) (-6.5948, 114.4321) knots 0 0 0 1 2 2 2
  line L245 (-6.5948, 114.4321) -> (-7.6584, 114.4321)
  line L246 (-7.6584, 114.4321) -> (-7.6584, 118.2876)
  line L247 (-7.6584, 118.2876) -> (-3.9936, 118.2876)
  line L248 (-3.9936, 118.2876) -> (-3.9936, 117.1835)
  line L249 (-3.9936, 117.1835) -> (-6.5081, 117.1835)
  line L250 (-6.5081, 117.1835) -> (-6.5081, 115.7789)
  spline S33 degree 2 poles (-6.5081, 115.7789) (-6.3347, 115.9292) (-5.8491, 116.091) (-5.6121, 116.091) knots 0 0 0 1 2 2 2
  spline S34 degree 2 poles (-5.6121, 116.091) (-4.7451, 116.091) (-3.7913, 114.9697) (-3.7913, 113.9523) knots 0 0 0 1 2 2 2
  line L251 (-3.7913, 113.9523) -> (-3.7913, 113.3627)
  spline S35 degree 2 poles (-3.7913, 113.3627) (-3.7913, 112.3396) (-4.8491, 111.2182) (-5.8087, 111.2182) knots 0 0 0 1 2 2 2
  line L252 (-8.3467, 86.4853) -> (-8.3467, 87.6678)
  line L253 (-8.3467, 87.6678) -> (-5.7703, 93.25)
  line L254 (-5.7703, 93.25) -> (-4.3434, 93.25)
  line L255 (-4.3434, 93.25) -> (-6.8471, 87.7339)
  line L256 (-6.8471, 87.7339) -> (-3.0948, 87.7339)
  line L257 (-3.0948, 87.7339) -> (-3.0948, 86.4853)
  line L258 (-3.0948, 86.4853) -> (-8.3467, 86.4853)
  line L259 (-5.004, 85.25) -> (-5.004, 89.9602)
  line L260 (-5.004, 89.9602) -> (-3.7026, 89.9602)
  line L261 (-3.7026, 89.9602) -> (-3.7026, 85.25)
  line L262 (-3.7026, 85.25) -> (-5.004, 85.25)
  spline S36 degree 2 poles (-5.852, 60.1806) (-6.459, 60.1806) (-7.4012, 60.6257) (-7.9618, 61.4697) (-8.0197, 62.065) knots 0 0 0 1 2 3 3 3
  line L263 (-8.0197, 62.065) -> (-6.8347, 62.065)
  spline S37 degree 2 poles (-6.8347, 62.065) (-6.7769, 61.6777) (-6.2971, 61.2905) (-5.9214, 61.2905) knots 0 0 0 1 2 2 2
  spline S38 degree 2 poles (-5.9214, 61.2905) (-5.4879, 61.2905) (-5.0197, 61.7645) (-5.0197, 62.1864) knots 0 0 0 1 2 2 2
  line L264 (-5.0197, 62.1864) -> (-5.0197, 62.3714)
  spline S39 degree 2 poles (-5.0197, 62.3714) (-5.0197, 62.8338) (-5.4358, 63.3425) (-5.8231, 63.3425) knots 0 0 0 1 2 2 2
  line L265 (-5.8231, 63.3425) -> (-6.3723, 63.3425)
  line L266 (-6.3723, 63.3425) -> (-6.3723, 64.4465)
  line L267 (-6.3723, 64.4465) -> (-5.8231, 64.4465)
  spline S40 degree 2 poles (-5.8231, 64.4465) (-5.4936, 64.4465) (-5.1353, 64.8801) (-5.1353, 65.2731) knots 0 0 0 1 2 2 2
  line L268 (-5.1353, 65.2731) -> (-5.1353, 65.4408)
  spline S41 degree 2 poles (-5.1353, 65.4408) (-5.1353, 65.8107) (-5.5225, 66.2095) (-5.8809, 66.2095) knots 0 0 0 1 2 2 2
  spline S42 degree 2 poles (-5.8809, 66.2095) (-6.1988, 66.2095) (-6.6439, 65.7991) (-6.7249, 65.3887) knots 0 0 0 1 2 2 2
  line L269 (-6.7249, 65.3887) -> (-7.904, 65.3887)
  spline S43 degree 2 poles (-7.904, 65.3887) (-7.7884, 66.3136) (-6.6786, 67.3251) (-5.852, 67.3251) knots 0 0 0 1 2 2 2
  spline S44 degree 2 poles (-5.852, 67.3251) (-4.9329, 67.3251) (-3.9329, 66.3772) (-3.9329, 65.5043) knots 0 0 0 1 2 2 2
  line L270 (-3.9329, 65.5043) -> (-3.9329, 65.3367)
  spline S45 degree 2 poles (-3.9329, 65.3367) (-3.9329, 64.8338) (-4.4647, 64.0882) (-4.9503, 63.9032) knots 0 0 0 1 2 2 2
  spline S46 degree 2 poles (-4.9503, 63.9032) (-4.4127, 63.7876) (-3.8173, 62.9321) (-3.8173, 62.2731) knots 0 0 0 1 2 2 2
  line L271 (-3.8173, 62.2731) -> (-3.8173, 62.1113)
  spline S47 degree 2 poles (-3.8173, 62.1113) (-3.8173, 61.1864) (-4.8809, 60.1806) (-5.852, 60.1806) knots 0 0 0 1 2 2 2
  line L272 (-7.7827, 34.7124) -> (-7.7827, 35.7355)
  line L273 (-7.7827, 35.7355) -> (-5.3607, 38.9379)
  spline S48 degree 2 poles (-5.3607, 38.9379) (-5.1699, 39.1864) (-4.9618, 39.7124) (-4.9618, 39.9379) knots 0 0 0 1 2 2 2
  line L274 (-4.9618, 39.9379) -> (-4.9618, 39.9436)
  spline S49 degree 2 poles (-4.9618, 39.9436) (-4.9618, 40.2962) (-5.3954, 40.6835) (-5.7884, 40.6835) knots 0 0 0 1 2 2 2
  spline S50 degree 2 poles (-5.7884, 40.6835) (-6.1584, 40.6835) (-6.6324, 40.2153) (-6.6844, 39.7876) knots 0 0 0 1 2 2 2
  line L275 (-6.6844, 39.7876) -> (-6.6844, 39.7818)
  line L276 (-6.6844, 39.7818) -> (-7.8694, 39.7818)
  line L277 (-7.8694, 39.7818) -> (-7.8694, 39.7876)
  spline S51 degree 2 poles (-7.8694, 39.7876) (-7.7653, 40.7413) (-6.6671, 41.7876) (-5.7942, 41.7876) knots 0 0 0 1 2 2 2
  spline S52 degree 2 poles (-5.7942, 41.7876) (-4.8289, 41.7876) (-3.7769, 40.8338) (-3.7769, 39.961) knots 0 0 0 1 2 2 2
  line L278 (-3.7769, 39.961) -> (-3.7769, 39.9552)
  spline S53 degree 2 poles (-3.7769, 39.9552) (-3.7769, 39.5332) (-4.0948, 38.6546) (-4.3838, 38.2789) knots 0 0 0 1 2 2 2
  line L279 (-4.3838, 38.2789) -> (-6.2566, 35.8165)
  line L280 (-6.2566, 35.8165) -> (-3.7364, 35.8165)
  line L281 (-3.7364, 35.8165) -> (-3.7364, 34.7124)
  line L282 (-3.7364, 34.7124) -> (-7.7827, 34.7124)
  line L283 (-4.9763, 16.25) -> (-4.9763, 9.25)
  line L284 (-4.9763, 9.25) -> (-6.1266, 9.25)
  line L285 (-6.1266, 9.25) -> (-6.1266, 14.9436)
  line L286 (-6.1266, 14.9436) -> (-7.0514, 14.4754)
  line L287 (-7.0514, 14.4754) -> (-7.0514, 15.6835)
  line L288 (-7.0514, 15.6835) -> (-6.0341, 16.25)
  line L289 (-6.0341, 16.25) -> (-4.9763, 16.25)
  line L290 (10.0929, -8.85) -> (12.3848, -2.75)
  line L291 (12.3848, -2.75) -> (13.1152, -2.75)
  line L292 (13.1152, -2.75) -> (15.4071, -8.85)
  line L293 (15.4071, -8.85) -> (14.3291, -8.85)
  line L294 (14.3291, -8.85) -> (12.7475, -4.3065)
  line L295 (12.7475, -4.3065) -> (11.1759, -8.85)
  line L296 (11.1759, -8.85) -> (10.0929, -8.85)
  line L297 (11.1709, -7.6915) -> (11.1709, -6.7294)
  line L298 (11.1709, -6.7294) -> (14.3795, -6.7294)
  line L299 (14.3795, -6.7294) -> (14.3795, -7.6915)
  line L300 (14.3795, -7.6915) -> (11.1709, -7.6915)
  line L301 (36.696, -8.85) -> (36.696, -7.898)
  line L302 (36.696, -7.898) -> (38.4943, -7.898)
  spline S54 degree 2 poles (38.4943, -7.898) (39.0333, -7.898) (39.532, -7.4497) (39.532, -7.0618) knots 0 0 0 1 2 2 2
  line L303 (39.532, -7.0618) -> (39.532, -7.0517)
  spline S55 degree 2 poles (39.532, -7.0517) (39.532, -6.6488) (39.0736, -6.1904) (38.6001, -6.1904) knots 0 0 0 1 2 2 2
  line L304 (38.6001, -6.1904) -> (36.696, -6.1904)
  line L305 (36.696, -6.1904) -> (36.696, -5.2484)
  line L306 (36.696, -5.2484) -> (38.6001, -5.2484)
  spline S56 degree 2 poles (38.6001, -5.2484) (39.0131, -5.2484) (39.4514, -4.8404) (39.4514, -4.4626) knots 0 0 0 1 2 2 2
  spline S57 degree 2 poles (39.4514, -4.4626) (39.4514, -4.0899) (38.9879, -3.697) (38.5396, -3.697) knots 0 0 0 1 2 2 2
  line L307 (38.5396, -3.697) -> (36.696, -3.697)
  line L308 (36.696, -3.697) -> (36.696, -2.75)
  line L309 (36.696, -2.75) -> (38.6353, -2.75)
  spline S58 degree 2 poles (38.6353, -2.75) (39.537, -2.75) (40.4638, -3.6315) (40.4638, -4.4022) knots 0 0 0 1 2 2 2
  spline S59 degree 2 poles (40.4638, -4.4022) (40.4638, -4.8958) (39.8846, -5.6212) (39.3103, -5.7219) knots 0 0 0 1 2 2 2
  spline S60 degree 2 poles (39.3103, -5.7219) (39.8946, -5.8076) (40.5394, -6.5984) (40.5394, -7.1777) knots 0 0 0 1 2 2 2
  line L310 (40.5394, -7.1777) -> (40.5394, -7.1877)
  spline S61 degree 2 poles (40.5394, -7.1877) (40.5394, -7.9584) (39.5672, -8.85) (38.7059, -8.85) knots 0 0 0 1 2 2 2
  line L311 (38.7059, -8.85) -> (36.696, -8.85)
  line L312 (36.1923, -8.85) -> (36.1923, -2.75)
  line L313 (36.1923, -2.75) -> (37.1947, -2.75)
  line L314 (37.1947, -2.75) -> (37.1947, -8.85)
  line L315 (37.1947, -8.85) -> (36.1923, -8.85)
  spline S62 degree 2 poles (63.6593, 212.9104) (64.3242, 212.9104) (65.2964, 212.3614) (65.8203, 211.3389) (65.8203, 210.6387) knots 0 0 0 1 2 3 3 3
  line L316 (65.8203, 210.6387) -> (65.8203, 208.9663)
  spline S63 degree 2 poles (65.8203, 208.9663) (65.8203, 208.2561) (65.2964, 207.2336) (64.3242, 206.6845) (63.6593, 206.6845) knots 0 0 0 1 2 3 3 3
  spline S64 degree 2 poles (63.6593, 206.6845) (63.1052, 206.6845) (62.2137, 207.158) (61.6243, 208.0395) (61.5135, 208.644) knots 0 0 0 1 2 3 3 3
  line L317 (61.5135, 208.644) -> (62.5461, 208.644)
  spline S65 degree 2 poles (62.5461, 208.644) (62.6217, 208.3417) (62.9491, 207.9136) (63.3974, 207.6768) (63.6593, 207.6768) knots 0 0 0 1 2 3 3 3
  spline S66 degree 2 poles (63.6593, 207.6768) (64.1782, 207.6768) (64.7877, 208.3669) (64.7877, 208.9663) knots 0 0 0 1 2 2 2
  line L318 (64.7877, 208.9663) -> (64.7877, 210.6387)
  spline S67 degree 2 poles (64.7877, 210.6387) (64.7877, 211.228) (64.1782, 211.9181) (63.6593, 211.9181) knots 0 0 0 1 2 2 2
  spline S68 degree 2 poles (63.6593, 211.9181) (63.2664, 211.9181) (62.6519, 211.4194) (62.5461, 210.951) knots 0 0 0 1 2 2 2
  line L319 (62.5461, 210.951) -> (61.5135, 210.951)
  spline S69 degree 2 poles (61.5135, 210.951) (61.6243, 211.5554) (62.2187, 212.437) (63.1052, 212.9104) (63.6593, 212.9104) knots 0 0 0 1 2 3 3 3
  line L320 (90.7763, 212.85) -> (90.7763, 211.8879)
  line L321 (90.7763, 211.8879) -> (89.3558, 211.8879)
  spline S70 degree 2 poles (89.3558, 211.8879) (88.7362, 211.8879) (88.0512, 211.2633) (88.0512, 210.6991) knots 0 0 0 1 2 2 2
  line L322 (88.0512, 210.6991) -> (88.0512, 208.9009)
  spline S71 degree 2 poles (88.0512, 208.9009) (88.0512, 208.3317) (88.7362, 207.7121) (89.3558, 207.7121) knots 0 0 0 1 2 2 2
  line L323 (89.3558, 207.7121) -> (90.7763, 207.7121)
  line L324 (90.7763, 207.7121) -> (90.7763, 206.75)
  line L325 (90.7763, 206.75) -> (89.381, 206.75)
  spline S72 degree 2 poles (89.381, 206.75) (88.2526, 206.75) (87.0185, 207.8934) (87.0185, 208.9361) knots 0 0 0 1 2 2 2
  line L326 (87.0185, 208.9361) -> (87.0185, 210.6639)
  spline S73 degree 2 poles (87.0185, 210.6639) (87.0185, 211.3338) (87.5626, 212.3161) (88.6153, 212.85) (89.386, 212.85) knots 0 0 0 1 2 3 3 3
  line L327 (89.386, 212.85) -> (90.7763, 212.85)
  line L328 (91.3555, 212.85) -> (91.3555, 206.75)
  line L329 (91.3555, 206.75) -> (90.3531, 206.75)
  line L330 (90.3531, 206.75) -> (90.3531, 212.85)
  line L331 (90.3531, 212.85) -> (91.3555, 212.85)
  line L332 (116.6037, 212.85) -> (116.6037, 206.75)
  line L333 (116.6037, 206.75) -> (115.6013, 206.75)
  line L334 (115.6013, 206.75) -> (115.6013, 212.85)
  line L335 (115.6013, 212.85) -> (116.6037, 212.85)
  line L336 (116.1906, 207.7121) -> (116.1906, 206.75)
  line L337 (116.1906, 206.75) -> (112.6042, 206.75)
  line L338 (112.6042, 206.75) -> (112.6042, 207.7121)
  line L339 (112.6042, 207.7121) -> (116.1906, 207.7121)
  line L340 (116.1906, 212.85) -> (116.1906, 211.8879)
  line L341 (116.1906, 211.8879) -> (112.6042, 211.8879)
  line L342 (112.6042, 211.8879) -> (112.6042, 212.85)
  line L343 (112.6042, 212.85) -> (116.1906, 212.85)
  line L344 (116.1906, 210.3012) -> (116.1906, 209.3391)
  line L345 (116.1906, 209.3391) -> (113.0626, 209.3441)
  line L346 (113.0626, 209.3441) -> (113.0626, 210.3012)
  line L347 (113.0626, 210.3012) -> (116.1906, 210.3012)
  line L348 (141.9374, 212.85) -> (141.9374, 206.75)
  line L349 (141.9374, 206.75) -> (140.9351, 206.75)
  line L350 (140.9351, 206.75) -> (140.9351, 212.85)
  line L351 (140.9351, 212.85) -> (141.9374, 212.85)
  line L352 (141.5194, 207.7121) -> (141.5194, 206.75)
  line L353 (141.5194, 206.75) -> (138.0185, 206.75)
  line L354 (138.0185, 206.75) -> (138.0185, 207.7121)
  line L355 (138.0185, 207.7121) -> (141.5194, 207.7121)
  line L356 (141.5194, 210.3516) -> (141.5194, 209.3945)
  line L357 (141.5194, 209.3945) -> (138.4769, 209.3945)
  line L358 (138.4769, 209.3945) -> (138.4769, 210.3516)
  line L359 (138.4769, 210.3516) -> (141.5194, 210.3516)
  line L360 (165.677, 209.5003) -> (163.5614, 209.5003)
  line L361 (163.5614, 209.5003) -> (163.5614, 210.6286)
  spline S74 degree 2 poles (163.5614, 210.6286) (163.5614, 211.3187) (164.1054, 212.3463) (165.0775, 212.9104) (165.7374, 212.9104) knots 0 0 0 1 2 3 3 3
  spline S75 degree 2 poles (165.7374, 212.9104) (166.3973, 212.9104) (167.3896, 212.3815) (167.9386, 211.4094) (167.9386, 210.7646) knots 0 0 0 1 2 3 3 3
  line L362 (167.9386, 210.7646) -> (167.9386, 208.9663)
  spline S76 degree 2 poles (167.9386, 208.9663) (167.9386, 208.2763) (167.3946, 207.2537) (166.4174, 206.6845) (165.7626, 206.6845) knots 0 0 0 1 2 3 3 3
  spline S77 degree 2 poles (165.7626, 206.6845) (165.2236, 206.6845) (164.327, 207.1379) (163.7175, 207.9539) (163.6117, 208.4979) knots 0 0 0 1 2 3 3 3
  line L363 (163.6117, 208.4979) -> (164.6947, 208.4979)
  spline S78 degree 2 poles (164.6947, 208.4979) (164.7955, 208.1151) (165.41, 207.697) (165.7626, 207.697) knots 0 0 0 1 2 2 2